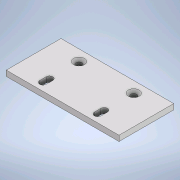
# Autodesk Inventor part: Motorhalterung_BT1
Saved by Autodesk Inventor 2020.1 (Build 241239000, 239)
## iProperties
Created: 2020-08-18
Part Number: Motorhalterung_BT1
Material: Generisch
Document SubType Name: Modeling
Designer: s5chfeis
Density: 1 g/cm^3
Appearance: Vorgabe
Author: s5chfeis
Autodesk Inventor part; units mm, degrees
ref_plane "YZ Plane" through (0, 0, 0) normal (1, 0, 0) x (0, 1, 0)
ref_plane "XZ Plane" through (0, 0, 0) normal (0, 1, 0) x (-1, 0, 0)
ref_plane "XY Plane" through (0, 0, 0) normal (0, 0, 1) x (1, 0, 0)
sketch "Skizze1" plane through (0, 0, 0) normal (0, 1, 0) x (-1, 0, 0)
  line L0 (0, 0) -> (-206, 0)
  line L1 (-206, 0) -> (-206, -100)
  line L2 (-206, -100) -> (0, -100)
  line L3 (0, -100) -> (0, 0)
  dimension "d0" = 206
  dimension "d1" = 100
  constraints: 8 end point, 2 parallel, 1 horizontal, 1 perpendicular
  measures "d0" distance of L2.end L1.end
  measures "d1" distance of L1.end L0.end
extrude "Extrusion1" add sketch "Skizze1" along normal blind 10
sketch "Skizze2" plane through (0, 10, 0) normal (0, 1, 0) x (1, 0, 0)
  line L0 (206, 100) -> (0, 100) construction
  line L1 (0, 100) -> (0, 20) construction
  line L2 (0, 100) -> (0, 0) construction
  line L3 (0, 100) -> (80, 100) construction
  line L4 (0, 20) -> (206, 20) construction
  line L5 (206, 20) -> (103, 20) construction
  line L6 (206, 20) -> (309, 20) construction
  line L7 (103, 20) -> (153, 20) construction
  line L8 (103, 20) -> (153, 20) construction
  line L9 (153, 20) -> (147, 20)
  line L10 (147, 20) -> (147, 26)
  line L11 (147, 26) -> (153, 26)
  line L12 (153, 26) -> (153, 20)
  line L13 (147, 20) -> (153, 20)
  line L14 (153, 20) -> (153, 14)
  line L15 (153, 14) -> (147, 14)
  line L16 (147, 14) -> (147, 20)
  arc A0 (147, 14) -> (153, 8) centre (153, 14) ccw
  arc A1 (153, 32) -> (147, 26) centre (153, 26) ccw
  line L17 (153, 8) -> (153, 32)
  line L18 (306, 20) -> (100, 20) construction
  line L19 (100, 20) -> (203, 20) construction
  line L20 (203, 20) -> (153, 20) construction
  line L21 (203, 20) -> (153, 20) construction
  line L22 (153, 20) -> (159, 20)
  line L23 (159, 20) -> (159, 26)
  line L24 (159, 26) -> (153, 26)
  line L25 (159, 20) -> (153, 20)
  line L26 (153, 14) -> (159, 14)
  line L27 (159, 14) -> (159, 20)
  arc A2 (153, 8) -> (159, 14) centre (153, 14) ccw
  arc A3 (159, 26) -> (153, 32) centre (153, 26) ccw
  line L28 (103, 100) -> (103, 20) construction
  line L29 (0, 0) -> (206, 0) construction
  line L30 (103, 100) -> (183, 100) construction
  line L31 (53, 20) -> (59, 20)
  line L32 (59, 20) -> (59, 26)
  line L33 (59, 26) -> (53, 26)
  line L34 (53, 26) -> (53, 20)
  line L35 (59, 20) -> (53, 20)
  line L36 (53, 20) -> (53, 14)
  line L37 (53, 14) -> (59, 14)
  line L38 (59, 14) -> (59, 20)
  arc A4 (53, 8) -> (59, 14) centre (53, 14) ccw
  arc A5 (59, 26) -> (53, 32) centre (53, 26) ccw
  line L39 (53, 8) -> (53, 32)
  line L40 (47, 20) -> (47, 26)
  line L41 (47, 26) -> (53, 26)
  line L42 (53, 20) -> (47, 20)
  line L43 (47, 20) -> (53, 20)
  line L44 (47, 14) -> (47, 20)
  line L45 (53, 14) -> (47, 14)
  arc A6 (53, 32) -> (47, 26) centre (53, 26) ccw
  arc A7 (47, 14) -> (53, 8) centre (53, 14) ccw
  dimension "d4" = 80
  dimension "d5" = 90
  dimension "d6" = 206
  dimension "d7" = 90
  dimension "d8" = 103
  dimension "d9" = 180
  dimension "d10" = 50
  dimension "d11" = 0
  dimension "d12" = 6
  dimension "d13" = 6
  dimension "d14" = 6
  dimension "d15" = 6
  dimension "d16" = 80
  dimension "d17" = 90
  constraints: 86 end point, 23 symmetric about line, 18 point on circle, 8 centre point, 8 coincident, 7 horizontal, 4 equal length, 4 parallel, 3 perpendicular, 2 collinear, 1 midpoint, 1 vertical, 7 other
  measures "d4" distance of L0.end L1.end
  measures "d5" angle of L1 L3
  measures "d6" distance of L1.end L4.end
  measures "d7" angle of L4 L1
  measures "d8" distance of L4.end L5.end
  measures "d9" angle of L5 L6
  measures "d10" distance of L5.end L7.end
  measures "d11" distance between parallel lines of L7 L8
  measures "d12" distance of L10.end L11.end
  measures "d13" distance of L9.end L10.end
  measures "d14" distance of L14.end L15.end
  measures "d15" distance of L13.end L14.end
  measures "d16" distance of L28.start L28.end
  measures "d17" angle of L28 L30
extrude "Extrusion2" cut sketch "Skizze2" against normal blind 10
sketch "Skizze4" plane through (0, 10, 0) normal (0, 1, 0) x (1, 0, 0)
  line L0 (0, 100) -> (0, 80) construction
  line L1 (0, 100) -> (0, 0) construction
  line L2 (0, 100) -> (20, 100) construction
  line L3 (0, 80) -> (206, 80) construction
  line L4 (0, 80) -> (103, 80) construction
  line L5 (103, 80) -> (53, 80) construction
  line L6 (53, 80) -> (153, 80) construction
  dimension "d24" = 20
  dimension "d25" = 90
  dimension "d26" = 206
  dimension "d27" = 90
  dimension "d28" = 50
  dimension "d29" = 100
  dimension "d30" = 0
  constraints: 12 end point, 2 coincident, 2 collinear, 2 perpendicular, 1 horizontal, 1 midpoint, 1 point on line
  measures "d24" distance of L0.start L0.end
  measures "d25" angle of L0 L2
  measures "d26" distance of L0.end L3.end
  measures "d27" angle of L3 L0
  measures "d28" distance of L4.end L5.end
  measures "d29" distance of L5.end L6.end
  measures "d30" distance between parallel lines of L6 L5
hole "Bohrung1" at (153, 10, -80) at (53, 10, -80) direction (0, -1, 0) diameter 11 end through all countersink diameter 20 countersink angle 90 clearance for "Flachkopfsenkschraube DIN EN ISO 2009" size "M10" standard "DIN"
